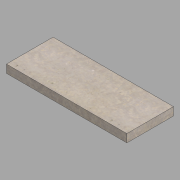
# Autodesk Inventor part: 23x60sawn
Saved by Autodesk Inventor 2022.2 (Build 262287000, 287)
## iProperties
Created: 2021-12-21
Part Number: 23x60sawn
Material: Limestone
Document SubType Name: Modeling
Designer: awelt
Mass: 232737 g
Surface Area: 21872.5 cm^2
Volume: 89514.3 cm^3
Density: 2.6 g/cm^3
Appearance: Kasota Gray
Author: awelt
Autodesk Inventor part; units mm, degrees
ref_plane "YZ Plane" through (0, 0, 0) normal (1, 0, 0) x (0, 1, 0)
ref_plane "XZ Plane" through (0, 0, 0) normal (0, 1, 0) x (-1, 0, 0)
ref_plane "XY Plane" through (0, 0, 0) normal (0, 0, 1) x (1, 0, 0)
sketch "Sketch1" plane through (0, 0, 0) normal (1, 0, 0) x (0, 1, 0)
  line L0 (0, 0) -> (101.6, 0)
  line L1 (101.6, 0) -> (101.6, 584.2)
  line L2 (101.6, 584.2) -> (0, 584.2)
  line L3 (0, 584.2) -> (0, 0)
  dimension "d0" = 101.6
  dimension "d1" = 584.2
  constraints: 8 end point, 2 parallel, 1 horizontal, 1 perpendicular
  measures "d0" distance of L2.end L1.end
  measures "d1" distance of L1.end L0.end
extrude "Extrusion1" add sketch "Sketch1" along normal blind 1508.125
body "Solid1"
